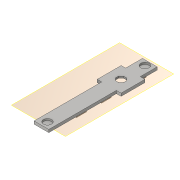
# Autodesk Inventor part: 02_Lensadapter
Saved by Autodesk Inventor 2016 (Build 200138000, 138)
## iProperties
Created: 2017-04-27
Part Number: 02_Lensadapter
Material: Generisch
Document SubType Name: Modeling
Designer: diederichbenedict
Density: 1 g/cm^3
Appearance: Vorgabe
Author: diederichbenedict
Autodesk Inventor part; units mm, degrees
note: some values were not read from the file. Chosen so that the rebuilt part matches the saved one: sketch regions of "Extrusion1".
ref_plane "YZ Plane" through (0, 0, 0) normal (1, 0, 0) x (0, 1, 0)
ref_plane "XZ Plane" through (0, 0, 0) normal (0, 1, 0) x (-1, 0, 0)
ref_plane "XY Plane" through (0, 0, 0) normal (0, 0, 1) x (1, 0, 0)
ref_plane "Arbeitsebene1" through (0, 0, 0) normal (0, 0, 1) x (1, 0, 0)
sketch "Skizze1" plane through (0, 0, 0) normal (0, 0, 1) x (1, 0, 0)
  circle A0 centre (-26.7746, 32.123) radius 1.5 construction
  circle A1 centre (15.7254, 11.123) radius 1.5 construction
  circle A2 centre (-26.2746, -24.877) radius 1.5 construction
  circle A3 centre (12.7254, -26.877) radius 1.5 construction
  circle A4 centre (12.7254, 30.123) radius 1.5 construction
  line L0 (11.0254, 3.323) -> (11.0254, -7.077) construction
  line L1 (11.0254, -7.077) -> (3.6254, -7.077) construction
  line L2 (3.6254, -7.077) -> (3.6254, 3.323) construction
  line L3 (3.6254, 3.323) -> (11.0254, 3.323) construction
  line L4 (3.6254, -32.077) -> (3.6254, -21.677) construction
  line L5 (3.6254, -21.677) -> (11.0254, -21.677) construction
  line L6 (11.0254, -21.677) -> (11.0254, -32.077) construction
  line L7 (11.0254, -32.077) -> (3.6254, -32.077) construction
  line L8 (11.0254, 27.923) -> (3.6254, 27.923) construction
  line L9 (3.6254, 27.923) -> (3.6254, 38.323) construction
  line L10 (3.6254, 38.323) -> (11.0254, 38.323) construction
  line L11 (11.0254, 38.323) -> (11.0254, 27.923) construction
  line L12 (-28.2746, 30.123) -> (-28.2746, -34.877) construction
  line L13 (-28.2746, -34.877) -> (-3.7746, -34.877) construction
  line L14 (-3.7746, -34.877) -> (-3.7746, -59.877) construction
  line L15 (-3.7746, -59.877) -> (10.8254, -59.877) construction
  line L16 (10.8254, -59.877) -> (10.8254, -34.877) construction
  line L17 (10.8254, -34.877) -> (20.2254, -34.877) construction
  line L18 (20.2254, -34.877) -> (20.2254, 39.123) construction
  line L19 (20.2254, 39.123) -> (10.8254, 39.123) construction
  line L20 (10.8254, 39.123) -> (10.8254, 49.123) construction
  line L21 (10.8254, 49.123) -> (-3.7746, 49.123) construction
  line L22 (-3.7746, 49.123) -> (-3.7746, 39.123) construction
  line L23 (-3.7746, 39.123) -> (-29.2746, 39.123) construction
  line L24 (-29.2746, 39.123) -> (-29.2746, 30.123) construction
  line L25 (-29.2746, 30.123) -> (-28.2746, 30.123) construction
  circle A5 centre (3.7254, 20.123) radius 7.5 construction
  line L26 (-3.7746, 49.123) -> (10.8254, 49.123) construction
  line L27 (10.8254, 49.123) -> (10.8254, -59.877) construction
  line L28 (10.8254, -59.877) -> (-3.7746, -59.877) construction
  line L29 (-3.7746, -59.877) -> (-3.7746, 49.123) construction
  line L30 (-3.7746, 49.123) -> (10.8254, 49.123)
  line L31 (10.8254, 49.123) -> (10.8254, -59.877)
  line L32 (10.8254, -59.877) -> (-3.7746, -59.877)
  line L33 (-3.7746, -59.877) -> (-3.7746, 49.123)
  circle A6 centre (3.7254, 44.123) radius 4.1 projected
  circle A7 centre (3.7254, -53.877) radius 4.1 projected
  line L34 (-8.2746, 32.123) -> (15.7254, 32.123)
  line L35 (15.7254, 32.123) -> (15.7254, 8.123)
  line L36 (15.7254, 8.123) -> (-8.2746, 8.123)
  line L37 (-8.2746, 8.123) -> (-8.2746, 32.123)
  line L38 (-8.2746, 32.123) -> (15.7254, 8.123) construction
  line L39 (15.7254, 32.123) -> (-8.2746, 8.123) construction
  circle A8 centre (3.7254, 20.123) radius 7.5
  circle A9 centre (3.7254, 20.123) radius 7.25
  line L40 (10.8254, 49.123) -> (10.9754, 49.123)
  line L41 (10.9754, 49.123) -> (10.9754, -59.877)
  line L42 (10.9754, -59.877) -> (10.8254, -59.877)
  line L43 (10.8254, -59.877) -> (10.8254, 49.123)
  point P0 (0, 0)
  dimension "d0" = 24
  dimension "d1" = 24
  dimension "d2" = 14.5
  dimension "d5" = 0.15
  constraints: 36 end point, 8 parallel, 4 horizontal, 4 perpendicular, 2 centre point, 2 coincident, 2 midpoint, 1 concentric
  measures "d0" distance of L35.end L36.end
  measures "d1" distance of L34.end L35.end
  measures "d2" diameter of A9
  measures "d5" distance of L15.end L41.end
extrude "Extrusion1" add sketch "Skizze1" along normal blind 1 contours L30 L31 L34 L33 | L40 L41 L34 L31 | L34 L31 A8 L33 | L33 L36 L37 L34 | L34 L41 A8 L31 | A8 L31 L36 L33 | A8 L31 A9 | A8 L41 A9 L31 | L34 L35 L36 L41 A8 | L36 L31 L32 L33 | A8 L41 L36 L31 | L31 A9 L41 A8 | A9 L31 | A8 L41 | L36 L41 L42 L31 | A6 | A7 picked at (10.8531, 19.7957)
sketch "Skizze2" plane through (0, 0, 0) normal (0, 0, -1) x (-1, 0, 0)
  circle A0 centre (26.7746, 32.123) radius 1.5 projected
  circle A1 centre (-15.7254, 11.123) radius 1.5 projected
  circle A2 centre (26.2746, -24.877) radius 1.5 projected
  circle A3 centre (-12.7254, -26.877) radius 1.5 projected
  circle A4 centre (-12.7254, 30.123) radius 1.5 projected
  line L0 (-11.0254, 3.323) -> (-11.0254, -7.077) projected
  line L1 (-11.0254, -7.077) -> (-3.6254, -7.077) projected
  line L2 (-3.6254, -7.077) -> (-3.6254, 3.323) projected
  line L3 (-3.6254, 3.323) -> (-11.0254, 3.323) projected
  line L4 (-3.6254, -32.077) -> (-3.6254, -21.677) projected
  line L5 (-3.6254, -21.677) -> (-11.0254, -21.677) projected
  line L6 (-11.0254, -21.677) -> (-11.0254, -32.077) projected
  line L7 (-11.0254, -32.077) -> (-3.6254, -32.077) projected
  line L8 (-11.0254, 27.923) -> (-3.6254, 27.923) projected
  line L9 (-3.6254, 27.923) -> (-3.6254, 38.323) projected
  line L10 (-3.6254, 38.323) -> (-11.0254, 38.323) projected
  line L11 (-11.0254, 38.323) -> (-11.0254, 27.923) projected
  line L12 (28.2746, 30.123) -> (28.2746, -34.877) projected
  line L13 (28.2746, -34.877) -> (3.7746, -34.877) projected
  line L14 (3.7746, -34.877) -> (3.7746, -59.877) projected
  line L15 (3.7746, -59.877) -> (-10.8254, -59.877) projected
  line L16 (-10.8254, -59.877) -> (-10.8254, -34.877) projected
  line L17 (-10.8254, -34.877) -> (-20.2254, -34.877) projected
  line L18 (-20.2254, -34.877) -> (-20.2254, 39.123) projected
  line L19 (-20.2254, 39.123) -> (-10.8254, 39.123) projected
  line L20 (-10.8254, 39.123) -> (-10.8254, 49.123) projected
  line L21 (-10.8254, 49.123) -> (3.7746, 49.123) projected
  line L22 (3.7746, 49.123) -> (3.7746, 39.123) projected
  line L23 (3.7746, 39.123) -> (29.2746, 39.123) projected
  line L24 (29.2746, 39.123) -> (29.2746, 30.123) projected
  line L25 (29.2746, 30.123) -> (28.2746, 30.123) projected
  circle A5 centre (-3.7254, 20.123) radius 7.5 projected
  line L26 (-3.8254, 38.123) -> (-3.8254, 28.123)
  line L27 (-3.8254, 28.123) -> (-10.8254, 28.123)
  line L28 (-10.8254, 28.123) -> (-10.8254, 38.123)
  line L29 (-10.8254, 38.123) -> (-3.8254, 38.123)
  line L30 (-3.8254, 3.123) -> (-3.8254, -6.877)
  line L31 (-3.8254, -6.877) -> (-10.8254, -6.877)
  line L32 (-10.8254, -6.877) -> (-10.8254, 3.123)
  line L33 (-10.8254, 3.123) -> (-3.8254, 3.123)
  line L34 (-10.8254, -21.877) -> (-3.8254, -21.877)
  line L35 (-3.8254, -21.877) -> (-3.8254, -31.877)
  line L36 (-3.8254, -31.877) -> (-10.8254, -31.877)
  line L37 (-10.8254, -31.877) -> (-10.8254, -21.877)
  point P0 (0, 0)
  dimension "d7" = 0.2
  dimension "d8" = 0.2
  dimension "d9" = 0.2
  constraints: 24 end point, 9 other
  measures "d7" distance between parallel lines of L9 L26
  measures "d8" distance between parallel lines of L2 L30
  measures "d9" distance between parallel lines of L5 L34
extrude "Extrusion2" add sketch "Skizze2" along normal blind 1 contours L26 L27 L28 L29 | L30 L31 L32 L33 | L34 L35 L36 L37
sketch "Skizze3" plane through (0, 0, 1) normal (0, 0, 1) x (1, 0, 0)
  circle A0 centre (3.7254, 20.123) radius 3.5 construction
  arc A1 (-0.3746, 17.023) -> (0.6254, 16.023) centre (0.6254, 17.023) ccw construction
  line L0 (0.6254, 16.023) -> (6.8254, 16.023) construction
  arc A2 (6.8254, 16.023) -> (7.8254, 17.023) centre (6.8254, 17.023) ccw construction
  line L1 (7.8254, 17.023) -> (7.8254, 18.7249) construction
  line L2 (7.8254, 18.7249) -> (9.8254, 18.7249) construction
  line L3 (9.8254, 19.2249) -> (9.8254, 18.7249) construction
  line L4 (7.8254, 19.2249) -> (9.8254, 19.2249) construction
  line L5 (7.8254, 19.2249) -> (7.8254, 21.021) construction
  line L6 (7.8254, 21.021) -> (9.8254, 21.021) construction
  line L7 (9.8254, 21.521) -> (9.8254, 21.021) construction
  line L8 (7.8254, 21.521) -> (9.8254, 21.521) construction
  line L9 (7.8254, 21.521) -> (7.8254, 23.223) construction
  arc A3 (7.8254, 23.223) -> (6.8254, 24.223) centre (6.8254, 23.223) ccw construction
  line L10 (6.8254, 24.223) -> (0.6254, 24.223) construction
  arc A4 (0.6254, 24.223) -> (-0.3746, 23.223) centre (0.6254, 23.223) ccw construction
  line L11 (-0.3746, 23.223) -> (-0.3746, 17.023) construction
  line L12 (10.9754, 49.123) -> (-3.7746, 49.123) projected
  line L13 (-3.7746, 49.123) -> (-3.7746, 32.123) projected
  line L14 (-3.7746, 32.123) -> (-8.2746, 32.123) projected
  line L15 (-8.2746, 32.123) -> (-8.2746, 8.123) projected
  line L16 (-8.2746, 8.123) -> (-3.7746, 8.123) projected
  line L17 (-3.7746, 8.123) -> (-3.7746, -59.877) projected
  line L18 (-3.7746, -59.877) -> (10.9754, -59.877) projected
  line L19 (10.9754, -59.877) -> (10.9754, 8.123) projected
  line L20 (10.9754, 8.123) -> (15.7254, 8.123) projected
  line L21 (15.7254, 8.123) -> (15.7254, 32.123) projected
  line L22 (15.7254, 32.123) -> (10.9754, 32.123) projected
  line L23 (10.9754, 32.123) -> (10.9754, 49.123) projected
  circle A5 centre (3.7254, 44.123) radius 4.1 projected
  circle A6 centre (3.7254, -53.877) radius 4.1 projected
  line L24 (-0.3246, 18.4454) -> (-0.3246, 21.8005)
  line L25 (-0.3246, 21.8005) -> (2.0478, 24.173)
  line L26 (2.0478, 24.173) -> (5.403, 24.173)
  line L27 (5.403, 24.173) -> (7.7754, 21.8005)
  line L28 (7.7754, 21.8005) -> (7.7754, 18.4454)
  line L29 (7.7754, 18.4454) -> (5.403, 16.073)
  line L30 (5.403, 16.073) -> (2.0478, 16.073)
  line L31 (2.0478, 16.073) -> (-0.3246, 18.4454)
  line L32 (-8.2746, 32.123) -> (-8.2746, 8.123) projected
  point P0 (0, 0)
  dimension "d16" = 8.1
  constraints: 16 end point, 1 parallel, 17 other
  measures "d16" distance between parallel lines of L28 L24
extrude "Extrusion3" add sketch "Skizze3" along normal blind 1.8
